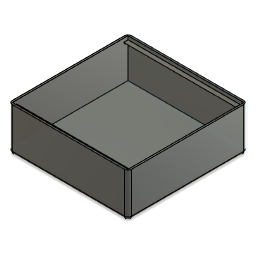
8x8 matrix box v3 (Autodesk Fusion 360 design; units mm, degrees)
Autodesk Fusion 360 part; units mm, degrees
note: some values were not read from the file. Chosen so that the rebuilt part matches the saved one: which pieces of a blend or face edit are solid.
sketch "Sketch1" plane through (0, 0, 0) normal (0, 1, 0) x (1, 0, 0)
  line L0 (33.75, 33.75) -> (-33.75, 33.75)
  line L1 (-33.75, 33.75) -> (-33.75, -33.75)
  line L2 (-33.75, -33.75) -> (33.75, -33.75)
  line L3 (33.75, -33.75) -> (33.75, 33.75)
  line L4 (33.75, 33.75) -> (-33.75, -33.75) construction
  line L5 (-33.75, 33.75) -> (33.75, -33.75) construction
  dimension "d1" = 67.5
  dimension "d2" = 67.5
  constraint horizontal L0
  constraint perpendicular L0 L1
  constraint parallel L0 L2
  constraint parallel L1 L3
  constraint coincident L4 origin
  constraint coincident L5 origin
  measures "d1" distance of L1.end L2.end
  measures "d2" distance of L0.end L1.end
extrude "Extrude1" add sketch "Sketch1" along normal blind 25
sketch "Sketch2" plane through (0, 25, 0) normal (0, 1, 0) x (-1, 0, 0)
  line L0 (-33.75, 33.75) -> (-33.75, -33.75)
  line L1 (-33.75, -33.75) -> (33.75, -33.75)
  line L2 (33.75, -33.75) -> (33.75, 33.75)
  line L3 (33.75, 33.75) -> (-33.75, 33.75)
  line L4 (-32.75, -32.75) -> (32.75, -32.75)
  line L5 (32.75, -32.75) -> (32.75, 32.75)
  line L6 (32.75, 32.75) -> (-32.75, 32.75)
  line L7 (-32.75, 32.75) -> (-32.75, -32.75)
  line L8 (-32.75, -32.75) -> (32.75, 32.75) construction
  line L9 (32.75, -32.75) -> (-32.75, 32.75) construction
  dimension "d5" = 65.5
  dimension "d6" = 65.5
  constraint horizontal L4
  constraint perpendicular L4 L5
  constraint parallel L4 L6
  constraint parallel L5 L7
  constraint coincident L8 origin
  constraint coincident L9 origin
  measures "d5" distance of L5.end L6.end
  measures "d6" distance of L4.end L5.end
extrude "Extrude2" cut sketch "Sketch2" against normal blind 22 contours L4 L5 L6 L7
sketch "Sketch3" plane through (0, 3, 0) normal (0, 1, 0) x (-1, 0, 0)
  line L0 (-32.75, 32.75) -> (-32.75, -32.75)
  line L1 (-32.75, -32.75) -> (32.75, -32.75)
  line L2 (32.75, -32.75) -> (32.75, 32.75)
  line L3 (32.75, 32.75) -> (-32.75, 32.75)
ref_plane "WorkPlane1" through (0, 22, 0) normal (0, 1, 0) x (-1, 0, 0)
sketch "Sketch4" plane through (0, 22, 0) normal (0, 1, 0) x (1, 0, 0)
ref_plane "WorkPlane2" through (0, 23, 0) normal (0, 1, 0) x (-1, 0, 0)
sketch "Sketch5" plane through (0, 23, 0) normal (0, 1, 0) x (1, 0, 0)
  line L0 (32.8932, 32.8932) -> (-32.8932, 32.8932)
  line L1 (-32.8932, 32.8932) -> (-32.8932, -32.8932)
  line L2 (-32.8932, -32.8932) -> (32.8932, -32.8932)
  line L3 (32.8932, -32.8932) -> (32.8932, 32.8932)
  line L4 (32.8932, 32.8932) -> (-32.8932, -32.8932) construction
  line L5 (-32.8932, 32.8932) -> (32.8932, -32.8932) construction
  constraint horizontal L0
  constraint perpendicular L0 L1
  constraint parallel L0 L2
  constraint parallel L1 L3
  constraint coincident L4 origin
  constraint coincident L5 origin
extrude "Extrude3" add sketch "Sketch5" against normal blind 2
sketch "Sketch6" plane through (0, 23, 0) normal (0, 1, 0) x (-1, 0, 0)
  line L0 (-32.75, -30.2083) -> (32.75, -30.2083)
  line L1 (32.75, -30.2083) -> (32.75, 30.2083)
  line L2 (32.75, 30.2083) -> (-32.75, 30.2083)
  line L3 (-32.75, 30.2083) -> (-32.75, -30.2083)
  line L4 (-32.75, -30.2083) -> (32.75, 30.2083) construction
  line L5 (32.75, -30.2083) -> (-32.75, 30.2083) construction
  line L6 (-32.75, -32.75) -> (32.75, -32.75)
  line L7 (32.75, -32.75) -> (32.75, 32.75)
  line L8 (32.75, 32.75) -> (-32.75, 32.75)
  line L9 (-32.75, 32.75) -> (-32.75, -32.75)
  constraint horizontal L0
  constraint perpendicular L0 L1
  constraint parallel L0 L2
  constraint parallel L1 L3
  constraint coincident L4 origin
  constraint coincident L5 origin
  constraint coincident L0.start L9
extrude "Extrude4" cut sketch "Sketch6" against normal blind 5 contours L0 L1 L2 L3 L7 L9
sketch "Sketch7" plane through (0, 0, -33.75) normal (0, 0, -1) x (-1, 0, 0)
  line L0 (-33.75, 0) -> (33.75, 0)
  line L1 (33.75, 0) -> (33.75, 25)
  line L2 (33.75, 25) -> (-33.75, 25)
  line L3 (-33.75, 25) -> (-33.75, 0)
sketch "Sketch8" plane through (0, 0, -32.75) normal (0, 0, 1) x (1, 0, 0)
  line L0 (32.75, 21) -> (-32.75, 21)
  line L1 (-32.75, 21) -> (-32.75, 3)
  line L2 (-32.75, 3) -> (32.75, 3)
  line L3 (32.75, 3) -> (32.75, 21)
  line L4 (31, 3.5) -> (20.5, 3.5)
  line L5 (20.5, 3.5) -> (20.5, 8.5)
  line L6 (20.5, 8.5) -> (31, 8.5)
  line L7 (31, 8.5) -> (31, 3.5)
  constraint horizontal L4
  constraint vertical L5
  constraint horizontal L6
  constraint vertical L7
extrude "Extrude5" cut sketch "Sketch8" against normal blind 1 contours L4 L5 L6 L7
fillet "Fillet2" radius 2 8 edges at (33.75, 0, 0) (0, 0, -33.75) (-33.75, 0, 0) (0, 0, 33.75) (33.75, 12.5, 33.75) (-33.75, 12.5, 33.75) (-33.75, 12.5, -33.75) (33.75, 12.5, -33.75)
fillet "Fillet3" radius 3.5 2 edges at (0, 21, -30.2083) (0, 21, 30.2083)
